Autodesk Fusion 360 part; units mm, degrees
(part 2 of 2)
sketch "lid underside - led holder" plane through (0, 0, 14.5) normal (0, 0, -1) x (1, 0, 0) in component "lid"
  arc A0 (-36.8, -16) -> (-36, -16.8) centre (-36, -16) ccw
  line L0 (-36, -16.8) -> (36, -16.8)
  arc A1 (36, -16.8) -> (36.8, -16) centre (36, -16) ccw
  line L1 (36.8, -16) -> (36.8, -10.6213)
  line L2 (36.8, -10.6213) -> (36.6787, -10.5)
  line L3 (36.6787, -10.5) -> (36.6787, 10.5)
  line L4 (36.6787, 10.5) -> (36.8, 10.6213)
  line L5 (36.8, 10.6213) -> (36.8, 16)
  arc A2 (36.8, 16) -> (36, 16.8) centre (36, 16) ccw
  line L6 (36, 16.8) -> (-36, 16.8)
  arc A3 (-36, 16.8) -> (-36.8, 16) centre (-36, 16) ccw
  line L7 (-36.8, 16) -> (-36.8, 10.6213)
  line L8 (-36.8, 10.6213) -> (-36.6787, 10.5)
  line L9 (-36.6787, 10.5) -> (-36.6787, -10.5)
  line L10 (-36.6787, -10.5) -> (-36.8, -10.6213)
  line L11 (-36.8, -10.6213) -> (-36.8, -16)
  circle A4 centre (26.5, 11.5) radius 0.7 construction
  circle A5 centre (23.9348, 11.5) radius 0.7 construction
  circle A6 centre (21.3696, 11.5) radius 0.7 construction
  circle A7 centre (18.8043, 11.5) radius 0.7 construction
  circle A8 centre (16.2391, 11.5) radius 0.7 construction
  circle A9 centre (13.6739, 11.5) radius 0.7 construction
  circle A10 centre (11.1087, 11.5) radius 0.7 construction
  circle A11 centre (8.5435, 11.5) radius 0.7 construction
  circle A12 centre (5.9783, 11.5) radius 0.7 construction
  circle A13 centre (3.413, 11.5) radius 0.7 construction
  circle A14 centre (0.8478, 11.5) radius 0.7 construction
  circle A15 centre (-1.7174, 11.5) radius 0.7 construction
  circle A16 centre (-4.2826, 11.5) radius 0.7 construction
  circle A17 centre (-6.8478, 11.5) radius 0.7 construction
  circle A18 centre (-9.413, 11.5) radius 0.7 construction
  circle A19 centre (-11.9783, 11.5) radius 0.7 construction
  circle A20 centre (-14.5435, 11.5) radius 0.7 construction
  circle A21 centre (-17.1087, 11.5) radius 0.7 construction
  circle A22 centre (-19.6739, 11.5) radius 0.7 construction
  circle A23 centre (-22.2391, 11.5) radius 0.7 construction
  circle A24 centre (-24.8043, 11.5) radius 0.7 construction
  circle A25 centre (-27.3696, 11.5) radius 0.7 construction
  circle A26 centre (-29.9348, 11.5) radius 0.7 construction
  circle A27 centre (-32.5, 11.5) radius 0.7 construction
  circle A28 centre (26.5, 8.9444) radius 0.7 construction
  circle A29 centre (23.9348, 8.9444) radius 0.7 construction
  circle A30 centre (21.3696, 8.9444) radius 0.7 construction
  circle A31 centre (18.8043, 8.9444) radius 0.7 construction
  circle A32 centre (16.2391, 8.9444) radius 0.7 construction
  circle A33 centre (13.6739, 8.9444) radius 0.7 construction
  circle A34 centre (11.1087, 8.9444) radius 0.7 construction
  circle A35 centre (8.5435, 8.9444) radius 0.7 construction
  circle A36 centre (5.9783, 8.9444) radius 0.7 construction
  circle A37 centre (3.413, 8.9444) radius 0.7 construction
  circle A38 centre (0.8478, 8.9444) radius 0.7 construction
  circle A39 centre (-1.7174, 8.9444) radius 0.7 construction
  circle A40 centre (-4.2826, 8.9444) radius 0.7 construction
  circle A41 centre (-6.8478, 8.9444) radius 0.7 construction
  circle A42 centre (-9.413, 8.9444) radius 0.7 construction
  circle A43 centre (-11.9783, 8.9444) radius 0.7 construction
  circle A44 centre (-14.5435, 8.9444) radius 0.7 construction
  circle A45 centre (-17.1087, 8.9444) radius 0.7 construction
  circle A46 centre (-19.6739, 8.9444) radius 0.7 construction
  circle A47 centre (-22.2391, 8.9444) radius 0.7 construction
  circle A48 centre (-24.8043, 8.9444) radius 0.7 construction
  circle A49 centre (-27.3696, 8.9444) radius 0.7 construction
  circle A50 centre (-29.9348, 8.9444) radius 0.7 construction
  circle A51 centre (-32.5, 8.9444) radius 0.7 construction
  circle A52 centre (26.5, 6.3889) radius 0.7 construction
  circle A53 centre (23.9348, 6.3889) radius 0.7 construction
  circle A54 centre (21.3696, 6.3889) radius 0.7 construction
  circle A55 centre (18.8043, 6.3889) radius 0.7 construction
  circle A56 centre (16.2391, 6.3889) radius 0.7 construction
  circle A57 centre (13.6739, 6.3889) radius 0.7 construction
  circle A58 centre (11.1087, 6.3889) radius 0.7 construction
  circle A59 centre (8.5435, 6.3889) radius 0.7 construction
  circle A60 centre (5.9783, 6.3889) radius 0.7 construction
  circle A61 centre (3.413, 6.3889) radius 0.7 construction
  circle A62 centre (0.8478, 6.3889) radius 0.7 construction
  circle A63 centre (-1.7174, 6.3889) radius 0.7 construction
  circle A64 centre (-4.2826, 6.3889) radius 0.7 construction
  circle A65 centre (-6.8478, 6.3889) radius 0.7 construction
  circle A66 centre (-9.413, 6.3889) radius 0.7 construction
  circle A67 centre (-11.9783, 6.3889) radius 0.7 construction
  circle A68 centre (-14.5435, 6.3889) radius 0.7 construction
  circle A69 centre (-17.1087, 6.3889) radius 0.7 construction
  circle A70 centre (-19.6739, 6.3889) radius 0.7 construction
  circle A71 centre (-22.2391, 6.3889) radius 0.7 construction
  circle A72 centre (-24.8043, 6.3889) radius 0.7 construction
  circle A73 centre (-27.3696, 6.3889) radius 0.7 construction
  circle A74 centre (-29.9348, 6.3889) radius 0.7 construction
  circle A75 centre (-32.5, 6.3889) radius 0.7 construction
  circle A76 centre (26.5, 3.8333) radius 0.7 construction
  circle A77 centre (23.9348, 3.8333) radius 0.7 construction
  circle A78 centre (21.3696, 3.8333) radius 0.7 construction
  circle A79 centre (18.8043, 3.8333) radius 0.7 construction
  circle A80 centre (16.2391, 3.8333) radius 0.7 construction
  circle A81 centre (13.6739, 3.8333) radius 0.7 construction
  circle A82 centre (11.1087, 3.8333) radius 0.7 construction
  circle A83 centre (8.5435, 3.8333) radius 0.7 construction
  circle A84 centre (5.9783, 3.8333) radius 0.7 construction
  circle A85 centre (3.413, 3.8333) radius 0.7 construction
  circle A86 centre (0.8478, 3.8333) radius 0.7 construction
  circle A87 centre (-1.7174, 3.8333) radius 0.7 construction
  circle A88 centre (-4.2826, 3.8333) radius 0.7 construction
  circle A89 centre (-6.8478, 3.8333) radius 0.7 construction
  circle A90 centre (-9.413, 3.8333) radius 0.7 construction
  circle A91 centre (-11.9783, 3.8333) radius 0.7 construction
  circle A92 centre (-14.5435, 3.8333) radius 0.7 construction
  circle A93 centre (-17.1087, 3.8333) radius 0.7 construction
  circle A94 centre (-19.6739, 3.8333) radius 0.7 construction
  circle A95 centre (-22.2391, 3.8333) radius 0.7 construction
  circle A96 centre (-24.8043, 3.8333) radius 0.7 construction
  circle A97 centre (-27.3696, 3.8333) radius 0.7 construction
  circle A98 centre (-29.9348, 3.8333) radius 0.7 construction
  circle A99 centre (-32.5, 3.8333) radius 0.7 construction
  circle A100 centre (26.5, 1.2778) radius 0.7 construction
  circle A101 centre (23.9348, 1.2778) radius 0.7 construction
  circle A102 centre (21.3696, 1.2778) radius 0.7 construction
  circle A103 centre (18.8043, 1.2778) radius 0.7 construction
  circle A104 centre (16.2391, 1.2778) radius 0.7 construction
  circle A105 centre (13.6739, 1.2778) radius 0.7 construction
  circle A106 centre (11.1087, 1.2778) radius 0.7 construction
  circle A107 centre (8.5435, 1.2778) radius 0.7 construction
  circle A108 centre (5.9783, 1.2778) radius 0.7 construction
  circle A109 centre (3.413, 1.2778) radius 0.7 construction
  circle A110 centre (0.8478, 1.2778) radius 0.7 construction
  circle A111 centre (-1.7174, 1.2778) radius 0.7 construction
  circle A112 centre (-4.2826, 1.2778) radius 0.7 construction
  circle A113 centre (-6.8478, 1.2778) radius 0.7 construction
  circle A114 centre (-9.413, 1.2778) radius 0.7 construction
  circle A115 centre (-11.9783, 1.2778) radius 0.7 construction
  circle A116 centre (-14.5435, 1.2778) radius 0.7 construction
  circle A117 centre (-17.1087, 1.2778) radius 0.7 construction
  circle A118 centre (-19.6739, 1.2778) radius 0.7 construction
  circle A119 centre (-22.2391, 1.2778) radius 0.7 construction
  circle A120 centre (-24.8043, 1.2778) radius 0.7 construction
  circle A121 centre (-27.3696, 1.2778) radius 0.7 construction
  circle A122 centre (-29.9348, 1.2778) radius 0.7 construction
  circle A123 centre (-32.5, 1.2778) radius 0.7 construction
  circle A124 centre (26.5, -1.2778) radius 0.7 construction
  circle A125 centre (23.9348, -1.2778) radius 0.7 construction
  circle A126 centre (21.3696, -1.2778) radius 0.7 construction
  circle A127 centre (18.8043, -1.2778) radius 0.7 construction
  circle A128 centre (16.2391, -1.2778) radius 0.7 construction
  circle A129 centre (13.6739, -1.2778) radius 0.7 construction
  circle A130 centre (11.1087, -1.2778) radius 0.7 construction
  circle A131 centre (8.5435, -1.2778) radius 0.7 construction
  circle A132 centre (5.9783, -1.2778) radius 0.7 construction
  circle A133 centre (3.413, -1.2778) radius 0.7 construction
  circle A134 centre (0.8478, -1.2778) radius 0.7 construction
  circle A135 centre (-1.7174, -1.2778) radius 0.7 construction
  circle A136 centre (-4.2826, -1.2778) radius 0.7 construction
  circle A137 centre (-6.8478, -1.2778) radius 0.7 construction
  circle A138 centre (-9.413, -1.2778) radius 0.7 construction
  circle A139 centre (-11.9783, -1.2778) radius 0.7 construction
  circle A140 centre (-14.5435, -1.2778) radius 0.7 construction
  circle A141 centre (-17.1087, -1.2778) radius 0.7 construction
  circle A142 centre (-19.6739, -1.2778) radius 0.7 construction
  circle A143 centre (-22.2391, -1.2778) radius 0.7 construction
  circle A144 centre (-24.8043, -1.2778) radius 0.7 construction
  circle A145 centre (-27.3696, -1.2778) radius 0.7 construction
  circle A146 centre (-29.9348, -1.2778) radius 0.7 construction
  circle A147 centre (-32.5, -1.2778) radius 0.7 construction
  circle A148 centre (26.5, -3.8333) radius 0.7 construction
  circle A149 centre (23.9348, -3.8333) radius 0.7 construction
  circle A150 centre (21.3696, -3.8333) radius 0.7 construction
  circle A151 centre (18.8043, -3.8333) radius 0.7 construction
  circle A152 centre (16.2391, -3.8333) radius 0.7 construction
  circle A153 centre (13.6739, -3.8333) radius 0.7 construction
  circle A154 centre (11.1087, -3.8333) radius 0.7 construction
  circle A155 centre (8.5435, -3.8333) radius 0.7 construction
  circle A156 centre (5.9783, -3.8333) radius 0.7 construction
  circle A157 centre (3.413, -3.8333) radius 0.7 construction
  circle A158 centre (0.8478, -3.8333) radius 0.7 construction
  circle A159 centre (-1.7174, -3.8333) radius 0.7 construction
  circle A160 centre (-4.2826, -3.8333) radius 0.7 construction
  circle A161 centre (-6.8478, -3.8333) radius 0.7 construction
  circle A162 centre (-9.413, -3.8333) radius 0.7 construction
  circle A163 centre (-11.9783, -3.8333) radius 0.7 construction
  circle A164 centre (-14.5435, -3.8333) radius 0.7 construction
  circle A165 centre (-17.1087, -3.8333) radius 0.7 construction
  circle A166 centre (-19.6739, -3.8333) radius 0.7 construction
  circle A167 centre (-22.2391, -3.8333) radius 0.7 construction
  circle A168 centre (-24.8043, -3.8333) radius 0.7 construction
  circle A169 centre (-27.3696, -3.8333) radius 0.7 construction
  circle A170 centre (-29.9348, -3.8333) radius 0.7 construction
  circle A171 centre (-32.5, -3.8333) radius 0.7 construction
  circle A172 centre (26.5, -6.3889) radius 0.7 construction
  circle A173 centre (23.9348, -6.3889) radius 0.7 construction
  circle A174 centre (21.3696, -6.3889) radius 0.7 construction
  circle A175 centre (18.8043, -6.3889) radius 0.7 construction
  circle A176 centre (16.2391, -6.3889) radius 0.7 construction
  circle A177 centre (13.6739, -6.3889) radius 0.7 construction
  circle A178 centre (11.1087, -6.3889) radius 0.7 construction
  circle A179 centre (8.5435, -6.3889) radius 0.7 construction
  circle A180 centre (5.9783, -6.3889) radius 0.7 construction
  circle A181 centre (3.413, -6.3889) radius 0.7 construction
  circle A182 centre (0.8478, -6.3889) radius 0.7 construction
  circle A183 centre (-1.7174, -6.3889) radius 0.7 construction
  circle A184 centre (-4.2826, -6.3889) radius 0.7 construction
  circle A185 centre (-6.8478, -6.3889) radius 0.7 construction
  circle A186 centre (-9.413, -6.3889) radius 0.7 construction
  circle A187 centre (-11.9783, -6.3889) radius 0.7 construction
  circle A188 centre (-14.5435, -6.3889) radius 0.7 construction
  circle A189 centre (-17.1087, -6.3889) radius 0.7 construction
  circle A190 centre (-19.6739, -6.3889) radius 0.7 construction
  circle A191 centre (-22.2391, -6.3889) radius 0.7 construction
  circle A192 centre (-24.8043, -6.3889) radius 0.7 construction
  circle A193 centre (-27.3696, -6.3889) radius 0.7 construction
  circle A194 centre (-29.9348, -6.3889) radius 0.7 construction
  circle A195 centre (-32.5, -6.3889) radius 0.7 construction
  circle A196 centre (26.5, -8.9444) radius 0.7 construction
  circle A197 centre (23.9348, -8.9444) radius 0.7 construction
  circle A198 centre (21.3696, -8.9444) radius 0.7 construction
  circle A199 centre (18.8043, -8.9444) radius 0.7 construction
  circle A200 centre (16.2391, -8.9444) radius 0.7 construction
  circle A201 centre (13.6739, -8.9444) radius 0.7 construction
  circle A202 centre (11.1087, -8.9444) radius 0.7 construction
  circle A203 centre (8.5435, -8.9444) radius 0.7 construction
  circle A204 centre (5.9783, -8.9444) radius 0.7 construction
  circle A205 centre (3.413, -8.9444) radius 0.7 construction
  circle A206 centre (0.8478, -8.9444) radius 0.7 construction
  circle A207 centre (-1.7174, -8.9444) radius 0.7 construction
  circle A208 centre (-4.2826, -8.9444) radius 0.7 construction
  circle A209 centre (-6.8478, -8.9444) radius 0.7 construction
  circle A210 centre (-9.413, -8.9444) radius 0.7 construction
  circle A211 centre (-11.9783, -8.9444) radius 0.7 construction
  circle A212 centre (-14.5435, -8.9444) radius 0.7 construction
  circle A213 centre (-17.1087, -8.9444) radius 0.7 construction
  circle A214 centre (-19.6739, -8.9444) radius 0.7 construction
  circle A215 centre (-22.2391, -8.9444) radius 0.7 construction
  circle A216 centre (-24.8043, -8.9444) radius 0.7 construction
  circle A217 centre (-27.3696, -8.9444) radius 0.7 construction
  circle A218 centre (-29.9348, -8.9444) radius 0.7 construction
  circle A219 centre (-32.5, -8.9444) radius 0.7 construction
  circle A220 centre (26.5, -11.5) radius 0.7 construction
  circle A221 centre (23.9348, -11.5) radius 0.7 construction
  circle A222 centre (21.3696, -11.5) radius 0.7 construction
  circle A223 centre (18.8043, -11.5) radius 0.7 construction
  circle A224 centre (16.2391, -11.5) radius 0.7 construction
  circle A225 centre (13.6739, -11.5) radius 0.7 construction
  circle A226 centre (11.1087, -11.5) radius 0.7 construction
  circle A227 centre (8.5435, -11.5) radius 0.7 construction
  circle A228 centre (5.9783, -11.5) radius 0.7 construction
  circle A229 centre (3.413, -11.5) radius 0.7 construction
  circle A230 centre (0.8478, -11.5) radius 0.7 construction
  circle A231 centre (-1.7174, -11.5) radius 0.7 construction
  circle A232 centre (-4.2826, -11.5) radius 0.7 construction
  circle A233 centre (-6.8478, -11.5) radius 0.7 construction
  circle A234 centre (-9.413, -11.5) radius 0.7 construction
  circle A235 centre (-11.9783, -11.5) radius 0.7 construction
  circle A236 centre (-14.5435, -11.5) radius 0.7 construction
  circle A237 centre (-17.1087, -11.5) radius 0.7 construction
  circle A238 centre (-19.6739, -11.5) radius 0.7 construction
  circle A239 centre (-22.2391, -11.5) radius 0.7 construction
  circle A240 centre (-24.8043, -11.5) radius 0.7 construction
  circle A241 centre (-27.3696, -11.5) radius 0.7 construction
  circle A242 centre (-29.9348, -11.5) radius 0.7 construction
  circle A243 centre (-32.5, -11.5) radius 0.7 construction
  circle A244 centre (30, 13.1) radius 1.2 construction
  circle A245 centre (-36, 13.1) radius 1.2 construction
  circle A246 centre (30, -13.1) radius 1.2 construction
  circle A247 centre (-36, -13.1) radius 1.2 construction
  line L12 (-38, 15) -> (32, 15) construction
  line L13 (-38, -15) -> (-38, 15) construction
  line L14 (32, -15) -> (-38, -15) construction
  line L15 (32, 15) -> (32, -15) construction
  circle A248 centre (26.5, 0) radius 3.05
  dimension "d237" = 6.1
  measures "d237" diameter of A248
extrude "Extrude4''" cut sketch "ports - top" against normal through all contours A4 A5 A6 A7 L4 L5 L6 L7 A85 A86 A87 A153 A154 A155 | L7 A153 | L5 A85 | L7 A154 | L5 A86 | L7 A155 | L5 A87 | A107 | A108 | A109 | A129 | A130 | A131 picked at (-13.5099, -3.7579) picked at (-13.7428, 3.6882) picked at (-10.9447, -3.7579) picked at (-11.1775, 3.6882) picked at (-8.3937, -3.7441) picked at (-8.4188, 3.7139) bodies 28 in component "lid"
extrude "Extrude7" add sketch "lid underside - led holder" along normal blind 3.7 contours A248 bodies 28 in component "lid"
extrude "Extrude8" cut sketch "ports - top" against normal up to surface (5.2 mm away) contours A248 bodies 28 in component "lid"
component "CO2 Sensor" placed x (1, 0, 0) y (0, 1, 0) z (0, 0, 1) at (0, 0, 0)
component "Internals" placed x (1, 0, 0) y (0, 1, 0) z (0, 0, 1) at (-3, 0, 34) in component "CO2 Sensor"
component "Case" placed x (1, 0, 0) y (0, 1, 0) z (0, 0, 1) at (0, 0, 0) in component "CO2 Sensor"
component "Board" placed x (1, 0, 0) y (0, 1, 0) z (0, 0, 1) at (0, 0, -29.5) in component "Internals"
component "RGBLED" placed x (1, 0, 0) y (0, 1, 0) z (0, 0, 1) at (29.5, -0.2, -24.5) in component "Internals"
component "D1 Mini" placed x (-1, 0, 0) y (0, -1, 0) z (0, 0, 1) at (-17.35, 0, -25.29) in component "Internals"
component "SCD41" placed x (1, 0, 0) y (0, 1, 0) z (0, 0, 1) at (14.3, 0.05, -22.6) in component "Internals"
component "pin" placed x (1, 0, 0) y (0, 1, 0) z (0, 0, 1) at (0, 0, 0) in component "Internals"
component "base (3)" placed x (1, 0, 0) y (0, 1, 0) z (0, 0, 1) at (0, 0, 0) in component "Case"
component "lid" placed x (1, 0, 0) y (0, 1, 0) z (0, 0, 1) at (0, 0, 0) in component "Case"
component "base" placed x (1, 0, 0) y (0, 1, 0) z (0, 0, 1) at (0, 0, 0) in component "D1 Mini"
component "CPU" placed x (1, 0, 0) y (0, 1, 0) z (0, 0, 1) at (0, 0, 0) in component "D1 Mini"
component "USB port" placed x (1, 0, 0) y (0, 1, 0) z (0, 0, 1) at (0, 0, 0) in component "D1 Mini"
component "pins" placed x (1, 0, 0) y (0, 1, 0) z (0, 0, 1) at (0, 0, 0) in component "D1 Mini"
component "board" placed x (1, 0, 0) y (0, 1, 0) z (0, 0, 1) at (0, 0, 0) in component "SCD41"
component "sensor5" placed x (1, 0, 0) y (0, 1, 0) z (0, 0, 1) at (0, 0, 0) in component "SCD41"
component "connectort" placed x (1, 0, 0) y (0, 1, 0) z (0, 0, 1) at (0, 0, 0) in component "SCD41"
component "pins (1)" placed x (1, 0, 0) y (0, 1, 0) z (0, 0, 1) at (0, 0, 0) in component "SCD41"
component "base (1)" placed x (1, 0, 0) y (0, 1, 0) z (0, 0, 1) at (0, 0, 0) in component "CPU"
component "CPU (1)" placed x (1, 0, 0) y (0, 1, 0) z (0, 0, 1) at (0, 0, 0) in component "CPU"
component "LED" placed x (1, 0, 0) y (0, 1, 0) z (0, 0, 1) at (0, 0, 0) in component "CPU"
component "pin (1)" placed x (1, 0, 0) y (0, 1, 0) z (0, 0, 1) at (0, 0, -5.8) in component "pin"
component "shroud" placed x (1, 0, 0) y (0, 1, 0) z (0, 0, 1) at (0, 0, 0) in component "pin"
component "pin (2)" placed x (1, 0, 0) y (0, 1, 0) z (0, 0, 1) at (0, 0, 1.5) in component "pins"
component "pin (2)" placed x (1, 0, 0) y (0, 1, 0) z (0, 0, 1) at (2.565, 0, 1.5) in component "pins"
component "pin (2)" placed x (1, 0, 0) y (0, 1, 0) z (0, 0, 1) at (5.13, 0, 1.5) in component "pins"
component "pin (2)" placed x (1, 0, 0) y (0, 1, 0) z (0, 0, 1) at (7.695, 0, 1.5) in component "pins"
component "pin (2)" placed x (1, 0, 0) y (0, 1, 0) z (0, 0, 1) at (10.26, 0, 1.5) in component "pins"
component "pin (2)" placed x (1, 0, 0) y (0, 1, 0) z (0, 0, 1) at (12.825, 0, 1.5) in component "pins"
component "pin (2)" placed x (1, 0, 0) y (0, 1, 0) z (0, 0, 1) at (15.39, 0, 1.5) in component "pins"
component "pin (2)" placed x (1, 0, 0) y (0, 1, 0) z (0, 0, 1) at (17.955, 0, 1.5) in component "pins"
component "pin (2)" placed x (1, 0, 0) y (0, 1, 0) z (0, 0, 1) at (0, 23, 1.5) in component "pins"
component "pin (2)" placed x (1, 0, 0) y (0, 1, 0) z (0, 0, 1) at (2.565, 23, 1.5) in component "pins"
component "pin (2)" placed x (1, 0, 0) y (0, 1, 0) z (0, 0, 1) at (5.13, 23, 1.5) in component "pins"
component "pin (2)" placed x (1, 0, 0) y (0, 1, 0) z (0, 0, 1) at (7.695, 23, 1.5) in component "pins"
component "pin (2)" placed x (1, 0, 0) y (0, 1, 0) z (0, 0, 1) at (10.26, 23, 1.5) in component "pins"
component "pin (2)" placed x (1, 0, 0) y (0, 1, 0) z (0, 0, 1) at (12.825, 23, 1.5) in component "pins"
component "pin (2)" placed x (1, 0, 0) y (0, 1, 0) z (0, 0, 1) at (15.39, 23, 1.5) in component "pins"
component "pin (2)" placed x (1, 0, 0) y (0, 1, 0) z (0, 0, 1) at (17.955, 23, 1.5) in component "pins"
component "pin (1) (1)" placed x (1, 0, 0) y (0, 1, 0) z (0, 0, 1) at (-8.375, -11.5, -9.96) in component "pin (2)"
component "shroud (1)" placed x (1, 0, 0) y (0, 1, 0) z (0, 0, 1) at (-8.375, -11.5, -4.16) in component "pin (2)"
component "base (2)" placed x (1, 0, 0) y (0, 1, 0) z (0, 0, 1) at (0, 0, 0) in component "sensor5"
component "housing" placed x (1, 0, 0) y (0, 1, 0) z (0, 0, 1) at (0, 0, 0) in component "sensor5"
component "pin (3)" placed x (1, 0, 0) y (0, 1, 0) z (0, 0, 1) at (-7.85, 3.85, -2.65) in component "pins (1)"
component "pin (3)" placed x (1, 0, 0) y (0, 1, 0) z (0, 0, 1) at (-7.85, 1.285, -2.65) in component "pins (1)"
component "pin (3)" placed x (1, 0, 0) y (0, 1, 0) z (0, 0, 1) at (-7.85, -1.28, -2.65) in component "pins (1)"
component "pin (3)" placed x (1, 0, 0) y (0, 1, 0) z (0, 0, 1) at (-7.85, -3.845, -2.65) in component "pins (1)"
component "pin (1) (2)" placed x (1, 0, 0) y (0, 1, 0) z (0, 0, 1) at (0, 0, -5.8) in component "pin (3)"
component "shroud (2)" placed x (1, 0, 0) y (0, 1, 0) z (0, 0, 1) at (0, 0, 0) in component "pin (3)"
equation "boardLength = 70 mm"
equation "boardWidth = 30 mm"
equation "boardHeight = 1.5 mm"
equation "d4 = boardLength"
equation "d5 = boardWidth"
equation "d6 = boardHeight"
equation "boardPostHoleLength = 66 mm"
equation "boardPostHoleWidth = 26.2 mm"
equation "boardPostHoleDiameter = 2.4 mm"
equation "d15 = boardPostHoleLength"
equation "d16 = boardPostHoleWidth"
equation "d17 = boardPostHoleDiameter"
equation "d22 = boardPostHoleLength"
equation "d23 = boardPostHoleWidth"
equation "d59 = ( 20.1 / 8 ) * 1 mm"
equation "d60 = ( 20.1 / 8 ) * 1 mm"
equation "d59_1 = ( 20.1 / 8 ) * 1 mm"
equation "d60_1 = ( 20.1 / 8 ) * 1 mm"
equation "d115 = ( 3 * 2.565 ) * 1 mm"
equation "d59_2 = ( 20.1 / 8 ) * 1 mm"
equation "d60_2 = ( 20.1 / 8 ) * 1 mm"
equation "caseLength = 80 mm"
equation "caseWidth = 40 mm"
equation "caseHeight = 14 mm"
equation "caseShell = 1.5 mm"
equation "caseGap = 0.2 mm"
equation "d169 = caseLength"
equation "d170 = caseWidth"
equation "d171 = caseHeight"
equation "d175 = caseShell"
equation "d176 = caseWidth / 2"
equation "d177 = caseShell * 2"
equation "d182 = lidShell"
equation "d184 = -( caseShell + caseGap )"
equation "d185 = 2 * caseShell"
equation "d192 = caseShell"
equation "d197 = boardPostHoleDiameter + 1 mm"
equation "boardPostHeight = 3 mm"
equation "d199 = boardPostHeight"
equation "d201 = boardPostHoleDiameter - 0.2 mm"
equation "d208 = boardPostHoleLength"
equation "d209 = boardPostHoleWidth"
equation "boardPostOffset = 2.5 mm"
equation "d211 = boardPostOffset"
equation "d214 = -boardPostHoleLength"
equation "d215 = boardPostHoleWidth"
equation "d225 = ledBodyDiameter"
equation "lidShell = 2 mm"
equation "ledBodyLength = 5.7 mm"
equation "d232 = ledBodyLength + 1 mm"
equation "d233 = ledBodyLength - lidShell"
equation "d237 = ledBodyDiameter + 1 mm"
equation "ledBodyDiameter = 5.1 mm"
named bodies: "base", "LED", "pin", "pin (1)", "pin (2)", "pin (3)", "case", "post", "post (1)", "post (2)", "post (3)"
